Cyclone  Saw to Cyclone Hose Adapter (Autodesk Fusion 360 design; units mm, degrees)
Autodesk Fusion 360 part; units mm, degrees
sketch "Sketch1" plane through (0, 0, 0) normal (0, 0, 1) x (1, 0, 0)
  circle A0 centre (0, 0) radius 28.25
  circle A1 centre (0, 0) radius 25.75
  dimension "d1" = 56.5
  dimension "d7" = 51.5
  constraint coincident A0.centre A1.centre
  constraint concentric A0 A1
  measures "d1" diameter of A0
  measures "d7" diameter of A1
ref_plane "WorkPlane1" through (0, 0, 40) normal (0, 0, 1) x (1, 0, 0)
sketch "Sketch2" plane through (0, 0, 40) normal (0, 0, 1) x (1, 0, 0)
  circle A0 centre (0, 0) radius 29
  circle A1 centre (0, 0) radius 26.6
  dimension "d6" = 58
  dimension "d8" = 53.2
  constraint coincident A0.centre A1.centre
  measures "d6" diameter of A0
  measures "d8" diameter of A1
loft "Loft1" add profiles "Sketch1", "Sketch2" section 1 section 2
loft "Loft2" cut profiles "Sketch2", "Sketch1" section 1 contours A1 section 2 contours A1
sketch "Sketch3" plane through (0, 0, 40) normal (0, 0, 1) x (1, 0, 0)
  circle A0 centre (0, 0) radius 32
  circle A1 centre (0, 0) radius 26.6
  circle A2 centre (0, 0) radius 24.1
  dimension "d9" = 64
  dimension "d10" = 53.2
  dimension "d15" = 48.2
  constraint coincident A0.centre A1.centre
  constraint concentric A1 A2
  measures "d9" diameter of A0
  measures "d10" diameter of A1
  measures "d15" diameter of A2
extrude "Extrude1" add sketch "Sketch3" along normal blind 5 contours A0
extrude "Extrude2" add sketch "Sketch3" along normal blind 45 contours A1
